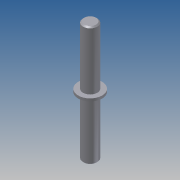
# Autodesk Inventor part: 23-225Z2
Saved by Autodesk Inventor 2011 SP2 (Build 150309200, 309)
## iProperties
Created: 2011-01-12
Part Number: 23-225Z2
Document SubType Name: Modeling
Designer: dc85560
Stock Number: 23-225Z2
Density: 8.08 g/cm^3
Material: Stainless Steel
Mass: 11.8336 g
Surface Area: 11.0169 cm^2
Volume: 1.46456 cm^3
Title: Concealed Hinge 40, Hinge Pin
Author: dc85560
Autodesk Inventor part; units mm, degrees
ref_plane "YZ Plane" through (0, 0, 0) normal (1, 0, 0) x (0, 1, 0)
ref_plane "XZ Plane" through (0, 0, 0) normal (0, 1, 0) x (-1, 0, 0)
ref_plane "XY Plane" through (0, 0, 0) normal (0, 0, 1) x (1, 0, 0)
sketch "Sketch1" plane through (0, 0, 0) normal (0, 0, 1) x (1, 0, 0)
  circle A0 centre (0, 0) radius 3
  dimension "d0" = 6
  constraints: 1 centre point, 1 coincident
  measures "d0" diameter of A0
extrude "Extrusion1" add sketch "Sketch1" against normal blind 50
ref_plane "Work Plane1" through (0, 0, -25) normal (0, 0, 1) x (1, 0, 0)
sketch "Sketch2" plane through (0, 0, -25) normal (0, 0, 1) x (1, 0, 0)
  circle A0 centre (0, 0) radius 3 projected
  circle A1 centre (0, 0) radius 3 projected
  circle A2 centre (0, 0) radius 5
  dimension "d3" = 10
  constraints: 1 centre point, 1 coincident
  measures "d3" diameter of A2
extrude "Extrusion2" add sketch "Sketch2" along normal mid plane 1.1
chamfer "Chamfer1" distance 0.5 angle 45 2 edges at (-3, 0, 0) (-3, 0, -50)
body "Solid1"
